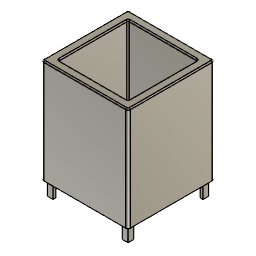
Drip-Through Holder-Top Section (Autodesk Fusion 360 design; units mm, degrees)
Autodesk Fusion 360 part; units mm, degrees
sketch "Sketch1" plane through (0, 0, 0) normal (0, 0, 1) x (1, 0, 0)
  line L0 (75, 75) -> (-75, 75)
  line L1 (-75, 75) -> (-75, -75)
  line L2 (-75, -75) -> (75, -75)
  line L3 (75, -75) -> (75, 75)
  line L4 (75, 75) -> (-75, -75) construction
  line L5 (-75, 75) -> (75, -75) construction
  line L6 (-50, 50) -> (-25, 50)
  line L7 (-25, 50) -> (-25, 25)
  line L8 (-25, 25) -> (-50, 25)
  line L9 (-50, 25) -> (-50, 50)
  line L10 (25, 50) -> (50, 50)
  line L11 (50, 50) -> (50, 25)
  line L12 (50, 25) -> (25, 25)
  line L13 (25, 25) -> (25, 50)
  line L14 (50, -50) -> (25, -50)
  line L15 (25, -50) -> (25, -25)
  line L16 (25, -25) -> (50, -25)
  line L17 (50, -25) -> (50, -50)
  line L18 (-25, -25) -> (-50, -25)
  line L19 (-50, -25) -> (-50, -50)
  line L20 (-50, -50) -> (-25, -50)
  line L21 (-25, -50) -> (-25, -25)
  line L22 (-60, -60) -> (60, -60)
  line L23 (60, -60) -> (60, 60)
  line L24 (60, 60) -> (-60, 60)
  line L25 (-60, 60) -> (-60, -60)
  dimension "d1" = 150
  dimension "d2" = 150
  constraint horizontal L0
  constraint perpendicular L0 L1
  constraint parallel L0 L2
  constraint parallel L1 L3
  constraint coincident L4 origin
  constraint coincident L5 origin
  constraint horizontal L6
  constraint vertical L7
  constraint horizontal L8
  constraint vertical L9
  constraint coincident L5 L7.end
  constraint coincident L5 L6.start
  constraint horizontal L10
  constraint vertical L11
  constraint horizontal L12
  constraint vertical L13
  constraint horizontal L14
  constraint vertical L15
  constraint horizontal L16
  constraint vertical L17
  constraint coincident L5 L15.end
  constraint coincident L5 L14.start
  constraint horizontal L18
  constraint vertical L19
  constraint horizontal L20
  constraint vertical L21
  constraint coincident L4 L19.end
  constraint coincident L4 L18.start
  constraint horizontal L22
  constraint vertical L23
  constraint horizontal L24
  constraint vertical L25
  constraint coincident L4 L23.end
  constraint coincident L4 L22.start
  measures "d1" distance of L1.end L2.end
  measures "d2" distance of L0.end L1.end
extrude "Extrude1" add sketch "Sketch1" along normal blind 180 contours L0 L1 L2 L3
extrude "Extrude2" add sketch "Sketch1" along normal blind 15 contours L22 L23 L24 L25
fillet "Fillet1" radius 2 4 edges at (-60, 60, 97.5) (-60, -60, 97.5) (60, -60, 97.5) (60, 60, 97.5)
fillet "Fillet2" radius 4 4 edges at (75, -75, 90) (75, 75, 90) (-75, 75, 90) (-75, -75, 90)
fillet "Fillet3" radius 2 8 edges at (-59.4142, 59.4142, 180) (0, 60, 180) (59.4142, 59.4142, 180) (60, 0, 180) (59.4142, -59.4142, 180) (0, -60, 180) (-59.4142, -59.4142, 180) (-60, 0, 180)
fillet "Fillet4" radius 1 32 edges at (-50, -25, 7.5) (-25, -50, 7.5) (-50, -50, 7.5) (-25, -25, 7.5) (50, -50, 7.5) (50, -25, 7.5) (25, -25, 7.5) (25, -50, 7.5) (-50, 25, 7.5) (-25, 25, 7.5) (-50, 50, 7.5) (-25, 50, 7.5) (50, 50, 7.5) (50, 25, 7.5) (25, 50, 7.5) (25, 25, 7.5) (-50, -37.5, 15) (-37.5, -50, 15) (-25, -37.5, 15) (-37.5, -25, 15) (25, 37.5, 15) (37.5, 25, 15) (37.5, -25, 15) (25, -37.5, 15) (37.5, -50, 15) (50, -37.5, 15) (50, 37.5, 15) (37.5, 50, 15) (-25, 37.5, 15) (-37.5, 25, 15) (-50, 37.5, 15) (-37.5, 50, 15)
fillet "Fillet5" radius 2 8 edges at (-59.4142, -59.4142, 15) (-60, 0, 15) (-59.4142, 59.4142, 15) (0, 60, 15) (59.4142, 59.4142, 15) (60, 0, 15) (59.4142, -59.4142, 15) (0, -60, 15)
sketch "Sketch2" plane through (0, 0, 0) normal (0, 0, 1) x (1, 0, 0)
  line L0 (70, 60) -> (70, 70)
  line L1 (70, 70) -> (60, 70)
  line L2 (60, 70) -> (60, 65)
  line L3 (60, 65) -> (65, 65)
  line L4 (65, 65) -> (65, 60)
  line L5 (65, 60) -> (70, 60)
  line L6 (70, -70) -> (70, -60)
  line L7 (70, -60) -> (65, -60)
  line L8 (65, -60) -> (65, -65)
  line L9 (65, -65) -> (60, -65)
  line L10 (60, -65) -> (60, -70)
  line L11 (60, -70) -> (70, -70)
  line L12 (-60, 65) -> (-60, 70)
  line L13 (-60, 70) -> (-70, 70)
  line L14 (-70, 70) -> (-70, 60)
  line L15 (-70, 60) -> (-65, 60)
  line L16 (-65, 60) -> (-65, 65)
  line L17 (-65, 65) -> (-60, 65)
  line L18 (-60, -70) -> (-60, -65)
  line L19 (-60, -65) -> (-65, -65)
  line L20 (-65, -65) -> (-65, -60)
  line L21 (-65, -60) -> (-70, -60)
  line L22 (-70, -60) -> (-70, -70)
  line L23 (-70, -70) -> (-60, -70)
  constraint vertical L0
  constraint perpendicular L0 L1
  constraint perpendicular L1 L2
  constraint perpendicular L2 L3
  constraint perpendicular L3 L4
  constraint perpendicular L0 L5
  constraint perpendicular L5 L6
  constraint perpendicular L6 L7
  constraint perpendicular L7 L8
  constraint perpendicular L8 L9
  constraint perpendicular L9 L10
  constraint perpendicular L6 L11
  constraint perpendicular L5 L12
  constraint perpendicular L12 L13
  constraint perpendicular L13 L14
  constraint perpendicular L14 L15
  constraint perpendicular L15 L16
  constraint perpendicular L12 L17
  constraint perpendicular L17 L18
  constraint perpendicular L18 L19
  constraint perpendicular L19 L20
  constraint perpendicular L20 L21
  constraint perpendicular L21 L22
  constraint perpendicular L18 L23
extrude "Extrude3" add sketch "Sketch2" against normal blind 25
move_body "Move1" bodies 1 to x (1, 0, 0) y (0, 1, 0) z (0, 0, 1) at (0, 0, 25)
fillet "Fillet6" radius 2 8 edges at (73.8284, 73.8284, 205) (0, 75, 205) (-73.8284, 73.8284, 205) (-75, 0, 205) (-73.8284, -73.8284, 205) (0, -75, 205) (73.8284, -73.8284, 205) (75, 0, 205)
sketch "Sketch3" plane through (0, 0, 25) normal (0, 0, -1) x (1, 0, 0)
  line L0 (70, -60) -> (70, -70)
  line L1 (70, -70) -> (60, -70)
  line L2 (60, -70) -> (60, -65)
  line L3 (60, -65) -> (65, -65)
  line L4 (65, -65) -> (65, -60)
  line L5 (65, -60) -> (70, -60)
  line L6 (-60, -65) -> (-60, -70)
  line L7 (-60, -70) -> (-70, -70)
  line L8 (-70, -70) -> (-70, -60)
  line L9 (-70, -60) -> (-65, -60)
  line L10 (-65, -60) -> (-65, -65)
  line L11 (-65, -65) -> (-60, -65)
  line L12 (70, 70) -> (70, 60)
  line L13 (70, 60) -> (65, 60)
  line L14 (65, 60) -> (65, 65)
  line L15 (65, 65) -> (60, 65)
  line L16 (60, 65) -> (60, 70)
  line L17 (60, 70) -> (70, 70)
  line L18 (-60, 70) -> (-60, 65)
  line L19 (-60, 65) -> (-65, 65)
  line L20 (-65, 65) -> (-65, 60)
  line L21 (-65, 60) -> (-70, 60)
  line L22 (-70, 60) -> (-70, 70)
  line L23 (-70, 70) -> (-60, 70)
  arc A0 (-71, 75) -> (-75, 71) centre (-71, 71) ccw
  line L24 (-75, 71) -> (-75, -71)
  arc A1 (-75, -71) -> (-71, -75) centre (-71, -71) ccw
  line L25 (-71, -75) -> (71, -75)
  arc A2 (71, -75) -> (75, -71) centre (71, -71) ccw
  line L26 (75, -71) -> (75, 71)
  arc A3 (75, 71) -> (71, 75) centre (71, 71) ccw
  line L27 (71, 75) -> (-71, 75)
  arc A4 (50, -26) -> (49, -25) centre (49, -26) ccw
  line L28 (50, -26) -> (50, -49)
  arc A5 (49, -50) -> (50, -49) centre (49, -49) ccw
  line L29 (49, -50) -> (26, -50)
  arc A6 (25, -49) -> (26, -50) centre (26, -49) ccw
  line L30 (25, -49) -> (25, -26)
  arc A7 (26, -25) -> (25, -26) centre (26, -26) ccw
  line L31 (26, -25) -> (49, -25)
  line L32 (-25, -26) -> (-25, -49)
  arc A8 (-26, -50) -> (-25, -49) centre (-26, -49) ccw
  line L33 (-26, -50) -> (-49, -50)
  arc A9 (-50, -49) -> (-49, -50) centre (-49, -49) ccw
  line L34 (-50, -49) -> (-50, -26)
  arc A10 (-49, -25) -> (-50, -26) centre (-49, -26) ccw
  line L35 (-49, -25) -> (-26, -25)
  arc A11 (-25, -26) -> (-26, -25) centre (-26, -26) ccw
  arc A12 (-26, 25) -> (-25, 26) centre (-26, 26) ccw
  line L36 (-26, 25) -> (-49, 25)
  arc A13 (-50, 26) -> (-49, 25) centre (-49, 26) ccw
  line L37 (-50, 26) -> (-50, 49)
  arc A14 (-49, 50) -> (-50, 49) centre (-49, 49) ccw
  line L38 (-49, 50) -> (-26, 50)
  arc A15 (-25, 49) -> (-26, 50) centre (-26, 49) ccw
  line L39 (-25, 49) -> (-25, 26)
  arc A16 (25, 26) -> (26, 25) centre (26, 26) ccw
  line L40 (25, 26) -> (25, 49)
  arc A17 (26, 50) -> (25, 49) centre (26, 49) ccw
  line L41 (26, 50) -> (49, 50)
  arc A18 (50, 49) -> (49, 50) centre (49, 49) ccw
  line L42 (50, 49) -> (50, 26)
  arc A19 (49, 25) -> (50, 26) centre (49, 26) ccw
  line L43 (49, 25) -> (26, 25)
  line L44 (-60, 60) -> (60, 60)
  line L45 (60, 60) -> (60, -60)
  line L46 (60, -60) -> (-60, -60)
  line L47 (-60, -60) -> (-60, 60)
  constraint horizontal L44
  constraint vertical L45
  constraint horizontal L46
  constraint vertical L47
extrude "Extrude4" add sketch "Sketch3" along normal blind 2.4 contours L44 L45 L46 L47
fillet "Fillet7" radius 2 4 edges at (60, 60, 23.8) (60, -60, 23.8) (-60, 60, 23.8) (-60, -60, 23.8)
